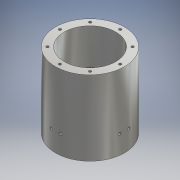
# Autodesk Inventor part: Enclosure
Saved by Autodesk Inventor 2016 (Build 200138000, 138)
## iProperties
Created: 2016-04-14
Part Number: Enclosure
Material: Generic
Document SubType Name: Modeling
Designer: Andres
Density: 1 g/cm^3
Appearance: Aluminum - Polished
Author: Andres
Autodesk Inventor part; units mm, degrees
ref_plane "YZ Plane" through (0, 0, 0) normal (1, 0, 0) x (0, 1, 0)
ref_plane "XZ Plane" through (0, 0, 0) normal (0, 1, 0) x (-1, 0, 0)
ref_plane "XY Plane" through (0, 0, 0) normal (0, 0, 1) x (1, 0, 0)
sketch "Sketch1" plane through (0, 0, 0) normal (0, 0, 1) x (1, 0, 0)
  circle A0 centre (0, 0) radius 40
  dimension "d32" = 80
  constraints: 1 centre point
  measures "d32" diameter of A0
extrude "Extrusion1" add sketch "Sketch1" along normal blind 87
sketch "Sketch2" plane through (0, 0, 87) normal (0, 0, 1) x (1, 0, 0)
  circle A0 centre (0, 0) radius 30
  point P0 (-21, 0)
  point P1 (0, 21)
  dimension "d86" = 60
  dimension "d87" = 21
  dimension "d88" = 21
  constraints: 1 centre point, 1 coincident, 1 horizontal alignment, 1 vertical alignment
  measures "d86" diameter of A0
  measures "d87" distance of point (0, 21) point (0, 0)
  measures "d88" distance of point (-21, 0) point (0, 0)
extrude "Extrusion2" cut sketch "Sketch2" against normal blind 42
sketch "Sketch3" plane through (0, 0, 45) normal (0, 0, 1) x (1, 0, 0)
  point P0 (0, 0)
sketch "Sketch4" plane through (0, 0, 0) normal (0, 0, -1) x (-1, 0, 0)
  circle A0 centre (0, 0) radius 11
  dimension "d8" = 22
  constraints: 1 centre point, 1 coincident
  measures "d8" diameter of A0
extrude "Extrusion3" cut sketch "Sketch4" against normal blind 10
sketch "Sketch5" plane through (0, 0, 10) normal (0, 0, -1) x (-1, 0, 0)
  circle A0 centre (0, 0) radius 1.25
  dimension "d11" = 2.5
  constraints: 1 centre point, 1 coincident
  measures "d11" diameter of A0
extrude "Extrusion4" cut sketch "Sketch5" against normal blind 35
ref_plane "Work Plane2" through (0, 0, 10) normal (0, 0, -1) x (-1, 0, 0)
sketch "Sketch9" plane through (0, 0, 0) normal (0, 0, -1) x (-1, 0, 0)
  point P0 (0, 0)
ref_plane "Work Plane7" through (20, -7.5, 0) normal (-1, 0, 0) x (0, 0, 1)
ref_plane "Work Plane8" through (-7.5, 20, 0) normal (0, -1, 0) x (1, 0, 0)
ref_plane "Work Plane9" through (-20, -7.5, 0) normal (1, 0, 0) x (0, 0, -1)
ref_plane "Work Plane10" through (-7.5, -20, 0) normal (0, 1, 0) x (1, 0, 0)
sketch "Sketch19" plane through (0, 0, 45) normal (0, 0, 1) x (1, 0, 0)
  circle A0 centre (0.0339, -24.2) radius 0.9
  circle A1 centre (24.2, 0) radius 0.9
  circle A2 centre (-24.2, 0) radius 0.9
  circle A3 centre (0.0339, 24.2) radius 0.9
  point P0 (0, 0)
  dimension "d89" = 1.8
  dimension "d90" = 24.2
  dimension "d91" = 1.8
  dimension "d92" = 24.2
  dimension "d93" = 1.8
  dimension "d94" = 24.2
  dimension "d95" = 1.8
  dimension "d96" = 24.2
  dimension "d97" = 34.2
  dimension "d98" = 34.2
  dimension "d100" = 48.4
  constraints: 4 centre point
  measures "d89" diameter of A0
  measures "d90" distance of A0.centre point (0, 0)
  measures "d91" diameter of A1
  measures "d92" distance of point (0, 0) A1.centre
  measures "d93" diameter of A2
  measures "d94" distance of A2.centre point (0, 0)
  measures "d95" diameter of A3
  measures "d96" distance of point (0, 0) A3.centre
  measures "d97" distance of A1.centre A3.centre
  measures "d98" distance of A1.centre A0.centre
  measures "d100" distance of A1.centre A2.centre
extrude "Extrusion14" cut sketch "Sketch19" against normal blind 10
sketch "Sketch20" plane through (0, 0, 10) normal (0, 0, -1) x (-1, 0, 0)
  circle A0 centre (-7.5, 0) radius 2.25
  circle A1 centre (0, -7.5) radius 2.25
  circle A2 centre (7.5, 0) radius 2.25
  circle A3 centre (0, 7.5) radius 2.25
  point P0 (0, 0)
  dimension "d103" = 4.5
  dimension "d104" = 4.5
  dimension "d105" = 4.5
  dimension "d106" = 4.5
  dimension "d109" = 7.5
  dimension "d111" = 7.5
  dimension "d112" = 7.5
  dimension "d114" = 7.5
  dimension "d115" = 7.5
  dimension "d116" = 7.5
  dimension "d117" = 7.5
  dimension "d118" = 7.5
  constraints: 4 centre point
  measures "d103" diameter of A0
  measures "d104" diameter of A1
  measures "d105" diameter of A2
  measures "d106" diameter of A3
  measures "d109" distance of point (0, 0) A2.centre
  measures "d111" distance of point (0, 0) A0.centre
  measures "d112" distance of point (0, 0) A1.centre
  measures "d114" distance of A3.centre point (0, 0)
  measures "d115" horizontal distance of A1.centre A2.centre
  measures "d116" horizontal distance of A0.centre A1.centre
  measures "d117" horizontal distance of A2.centre A3.centre
  measures "d118" horizontal distance of A1.centre A2.centre
extrude "Extrusion15" cut sketch "Sketch20" against normal blind 20
ref_plane "Work Plane11" through (-7.5, -30, 0) normal (0, 1, 0) x (1, 0, 0)
sketch "Sketch22" plane through (-7.5, -30, 0) normal (0, 1, 0) x (1, 0, 0)
  line L0 (-5, 0) -> (20, 0) projected
  line L1 (-5, -30) -> (-5, 0) projected
  line L2 (20, -30) -> (-5, -30) projected
  line L3 (20, 0) -> (20, -30) projected
  point P0 (7.5, 0)
extrude "Extrusion16" cut sketch "Sketch22" along normal mid plane 5
ref_plane "Work Plane12" through (30, -7.5, 0) normal (-1, 0, 0) x (0, 0, 1)
sketch "Sketch23" plane through (30, -7.5, 0) normal (-1, 0, 0) x (0, 0, 1)
  line L0 (0, -5) -> (0, 20) projected
  line L1 (29.9794, -5) -> (0, -5) projected
  line L2 (29.9794, 20) -> (29.9794, -5) projected
  line L3 (0, 20) -> (29.9794, 20) projected
  point P0 (0, 7.5)
extrude "Extrusion17" cut sketch "Sketch23" along normal mid plane 5
ref_plane "Work Plane13" through (-7.5, 30, 0) normal (0, -1, 0) x (1, 0, 0)
sketch "Sketch24" plane through (-7.5, 30, 0) normal (0, -1, 0) x (1, 0, 0)
  point P0 (7.5, 0)
sketch "Sketch25" plane through (-7.5, 30, 0) normal (0, -1, 0) x (1, 0, 0)
  line L0 (20, 0) -> (-5, 0) projected
  line L1 (20, 30) -> (20, 0) projected
  line L2 (-5, 30) -> (20, 30) projected
  line L3 (-5, 0) -> (-5, 30) projected
  point P0 (7.5, 0)
extrude "Extrusion18" cut sketch "Sketch25" along normal mid plane 5
ref_plane "Work Plane14" through (-30, -7.5, 0) normal (1, 0, 0) x (0, 0, -1)
sketch "Sketch26" plane through (-30, -7.5, 0) normal (1, 0, 0) x (0, 0, -1)
  line L0 (0, 20) -> (0, -5) projected
  line L1 (-29.7528, 20) -> (0, 20) projected
  line L2 (-29.7528, -5) -> (-29.7528, 20) projected
  line L3 (0, -5) -> (-29.7528, -5) projected
  point P0 (0, 7.5)
extrude "Extrusion19" cut sketch "Sketch26" along normal mid plane 5
ref_plane "Work Plane16" through (32.5, -7.5, 0) normal (-1, 0, 0) x (0, 0, 1)
sketch "Sketch27" plane through (32.5, -7.5, 0) normal (-1, 0, 0) x (0, 0, 1)
  circle A0 centre (21.9794, 2.25) radius 1.5
  line L0 (0, -5) -> (29.9794, -5) projected
  line L1 (29.9794, -5) -> (29.9794, 20) projected
  circle A1 centre (21.9794, 12.75) radius 1.5
  line L2 (29.9794, 20) -> (0, 20) projected
  point P0 (0, 7.5)
  dimension "d134" = 7.25
  dimension "d136" = 8
  dimension "d137" = 3
  dimension "d138" = 3
  dimension "d139" = 7.25
  dimension "d140" = 8
  constraints: 2 centre point
  measures "d134" distance from line of L0 A0.centre
  measures "d136" distance from line of L1 A0.centre
  measures "d137" diameter of A0
  measures "d138" diameter of A1
  measures "d139" distance from line of L2 A1.centre
  measures "d140" distance from line of L1 A1.centre
extrude "Extrusion20" cut sketch "Sketch27" against normal blind 7.5
ref_plane "Work Plane17" through (-7.5, -32.5, 0) normal (0, 1, 0) x (1, 0, 0)
sketch "Sketch29" plane through (-7.5, -32.5, 0) normal (0, 1, 0) x (1, 0, 0)
  line L0 (20, 0) -> (-5, 0) projected
  line L1 (20, -30) -> (20, 0) projected
  line L2 (-5, -30) -> (20, -30) projected
  line L3 (-5, 0) -> (-5, -30) projected
  circle A0 centre (2.25, -22) radius 1.5
  circle A1 centre (12.75, -22) radius 1.5
  point P0 (7.5, 0)
  dimension "d144" = 3
  dimension "d145" = 3
  dimension "d146" = 7.25
  dimension "d147" = 8
  dimension "d148" = 7.25
  dimension "d149" = 8
  constraints: 2 centre point
  measures "d144" diameter of A0
  measures "d145" diameter of A1
  measures "d146" distance from line of L3 A0.centre
  measures "d147" distance from line of L2 A0.centre
  measures "d148" distance from line of L1 A1.centre
  measures "d149" distance from line of L2 A1.centre
extrude "Extrusion21" cut sketch "Sketch29" against normal blind 7.5 contours A0 | A1
ref_plane "Work Plane18" through (-32.5, -7.5, 0) normal (1, 0, 0) x (0, 0, -1)
sketch "Sketch30" plane through (-32.5, -7.5, 0) normal (1, 0, 0) x (0, 0, -1)
  circle A0 centre (-21.7528, 12.75) radius 1.5
  circle A1 centre (-21.7528, 2.25) radius 1.5
  line L0 (-29.7528, 20) -> (-29.7528, -5) projected
  line L1 (0, 20) -> (-29.7528, 20) projected
  line L2 (-29.7528, -5) -> (0, -5) projected
  point P0 (0, 7.5)
  dimension "d153" = 3
  dimension "d154" = 3
  dimension "d155" = 8
  dimension "d156" = 8
  dimension "d157" = 7.25
  dimension "d158" = 7.25
  constraints: 2 centre point
  measures "d153" diameter of A0
  measures "d154" diameter of A1
  measures "d155" distance from line of L0 A0.centre
  measures "d156" distance from line of L0 A1.centre
  measures "d157" distance from line of L1 A0.centre
  measures "d158" distance from line of L2 A1.centre
extrude "Extrusion22" cut sketch "Sketch30" against normal blind 7.5
ref_plane "Work Plane19" through (-7.5, 32.5, 0) normal (0, -1, 0) x (1, 0, 0)
sketch "Sketch31" plane through (-7.5, 32.5, 0) normal (0, -1, 0) x (1, 0, 0)
  line L0 (-5, 0) -> (20, 0) projected
  line L1 (-5, 30) -> (-5, 0) projected
  line L2 (20, 30) -> (-5, 30) projected
  line L3 (20, 0) -> (20, 30) projected
  circle A0 centre (12.75, 22) radius 1.5
  circle A1 centre (2.25, 22) radius 1.5
  point P0 (7.5, 0)
  dimension "d162" = 3
  dimension "d163" = 8
  dimension "d164" = 8
  dimension "d165" = 7.25
  dimension "d166" = 7.25
  dimension "d167" = 3
  constraints: 2 centre point
  measures "d162" diameter of A1
  measures "d163" distance from line of L2 A0.centre
  measures "d164" distance from line of L2 A1.centre
  measures "d165" distance from line of L1 A1.centre
  measures "d166" distance from line of L3 A0.centre
  measures "d167" diameter of A0
extrude "Extrusion23" cut sketch "Sketch31" against normal blind 7.5 contours A0 | A1
ref_plane "Work Plane20" through (-7.5, 27.5, 0) normal (0, 1, 0) x (1, 0, 0)
sketch "Sketch32" plane through (-7.5, 27.5, 0) normal (0, 1, 0) x (1, 0, 0)
  circle A0 centre (12.75, -22) radius 1.5 projected
  circle A1 centre (2.25, -22) radius 1.5 projected
  point P0 (7.5, 0)
extrude "Extrusion24" cut sketch "Sketch32" against normal blind 5
ref_plane "Work Plane21" through (27.5, -7.5, 0) normal (1, 0, 0) x (0, 0, -1)
sketch "Sketch33" plane through (27.5, -7.5, 0) normal (1, 0, 0) x (0, 0, -1)
  circle A0 centre (-21.9794, 2.25) radius 1.5 projected
  circle A1 centre (-21.9794, 12.75) radius 1.5 projected
  point P0 (0, 7.5)
extrude "Extrusion25" cut sketch "Sketch33" against normal blind 5
ref_plane "Work Plane22" through (-7.5, -27.5, 0) normal (0, -1, 0) x (1, 0, 0)
sketch "Sketch34" plane through (-7.5, -27.5, 0) normal (0, -1, 0) x (1, 0, 0)
  circle A0 centre (12.75, 22) radius 1.5 projected
  circle A1 centre (2.25, 22) radius 1.5 projected
  point P0 (7.5, 0)
extrude "Extrusion26" cut sketch "Sketch34" against normal blind 5
ref_plane "Work Plane23" through (-27.5, -7.5, 0) normal (-1, 0, 0) x (0, 0, 1)
sketch "Sketch35" plane through (-27.5, -7.5, 0) normal (-1, 0, 0) x (0, 0, 1)
  circle A0 centre (21.7528, 2.25) radius 1.5 projected
  circle A1 centre (21.7528, 12.75) radius 1.5 projected
  point P0 (0, 7.5)
extrude "Extrusion27" cut sketch "Sketch35" against normal blind 5
sketch "Sketch36" plane through (0, 0, 87) normal (0, 0, 1) x (1, 0, 0)
  circle A0 centre (0, 0) radius 40 projected
  circle A1 centre (0, 35) radius 1.5
  line L0 (-12.5, 32.5) -> (12.5, 32.5) projected
  circle A2 centre (-24.7487, 24.7487) radius 1.5
  circle A3 centre (-35, 0) radius 1.5
  circle A4 centre (-24.7487, -24.7487) radius 1.5
  circle A5 centre (0, -35) radius 1.5
  circle A6 centre (24.7487, -24.7487) radius 1.5
  circle A7 centre (35, 0) radius 1.5
  circle A8 centre (24.7487, 24.7487) radius 1.5
  point P0 (0, 32.5)
  dimension "d182" = 3
  dimension "d183" = 35
  dimension "d186" = 360
  constraints: 8 centre point, 1 midpoint, 1 vertical alignment, 17 other
  measures "d182" diameter of A1
  measures "d183" distance of point (0, 0) A1.centre
extrude "Extrusion28" cut sketch "Sketch36" against normal blind 25 contours A1 | A2 | A3 | A4 | A5 | A6 | A7 | A8
body "Solid1"
